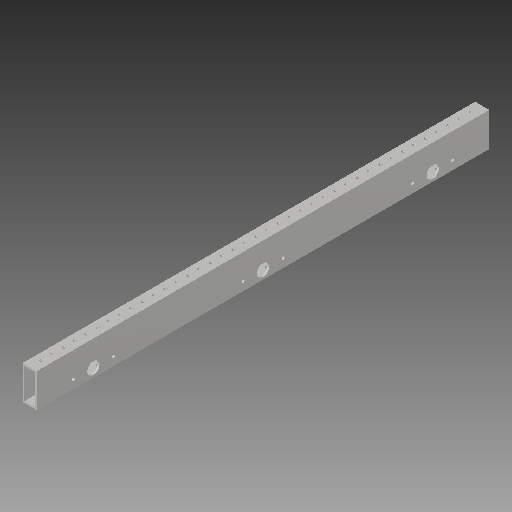
# Autodesk Inventor part: Side Extrusion
Saved by Autodesk Inventor 2019.4 (Build 234330000, 330)
## iProperties
Created: 2019-12-11
Part Number: Side Extrusion
Material: Aluminum 6061
Document SubType Name: Modeling
Designer: Mark
Mass: 988.046 g
Surface Area: 2508.19 cm^2
Volume: 365.943 cm^3
Density: 2.7 g/cm^3
Appearance: Aluminum - Flat
Author: Mark
Autodesk Inventor part; units mm, degrees
ref_plane "YZ Plane" through (0, 0, 0) normal (1, 0, 0) x (0, 1, 0)
ref_plane "XZ Plane" through (0, 0, 0) normal (0, 1, 0) x (-1, 0, 0)
ref_plane "XY Plane" through (0, 0, 0) normal (0, 0, 1) x (1, 0, 0)
sketch "Sketch1" plane through (0, 0, 0) normal (0, 0, 1) x (1, 0, 0)
  line L0 (-12.5, -30) -> (12.5, -30)
  line L1 (12.5, -30) -> (12.5, 30)
  line L2 (12.5, 30) -> (-12.5, 30)
  line L3 (-12.5, 30) -> (-12.5, -30)
  line L4 (-12.5, -30) -> (12.5, 30) construction
  line L5 (12.5, -30) -> (-12.5, 30) construction
  line L6 (-9.5, -27) -> (9.5, -27)
  line L7 (9.5, -27) -> (9.5, 27)
  line L8 (9.5, 27) -> (-9.5, 27)
  line L9 (-9.5, 27) -> (-9.5, -27)
  line L10 (-9.5, -27) -> (9.5, 27) construction
  line L11 (9.5, -27) -> (-9.5, 27) construction
  point P0 (0, 0)
  dimension "d0" = 25
  dimension "d1" = 60
  dimension "d2" = 19
  dimension "d3" = 54
  constraints: 24 end point, 4 midpoint, 4 parallel, 2 horizontal, 2 perpendicular
  measures "d0" distance of L2.end L1.end
  measures "d1" distance of L1.end L0.end
  measures "d2" distance of L8.end L7.end
  measures "d3" distance of L7.end L6.end
extrude "Extrusion1" add sketch "Sketch1" along normal blind 800
sketch "Sketch2" plane through (12.5, -30, 0) normal (1, 0, 0) x (0, 0, -1)
  circle A0 centre (-400, 15) radius 11
  circle A1 centre (-700, 15) radius 11
  circle A2 centre (-100, 15) radius 11
  line L0 (0, 60) -> (-800, 60) projected
  line L1 (-800, 0) -> (-800, 60) projected
  circle A3 centre (-700, 15) radius 35.5 construction
  circle A4 centre (-735.5, 15) radius 2.75
  circle A5 centre (-664.5, 15) radius 2.75
  line L2 (-700, 15) -> (-735.5, 15) construction
  line L3 (-700, 15) -> (-664.5, 15) construction
  line L4 (-400, 15) -> (-400, 60)
  circle A6 centre (-435.5, 15) radius 2.75
  line L5 (0, 0) -> (-800, 0) projected
  circle A7 centre (-64.5, 15) radius 2.75
  circle A8 centre (-135.5, 15) radius 2.75
  circle A9 centre (-364.5, 15) radius 2.75
  point P0 (0, 30)
  dimension "d6" = 22
  dimension "d7" = 22
  dimension "d8" = 22
  dimension "d9" = 45
  dimension "d10" = 45
  dimension "d11" = 45
  dimension "d12" = 400
  dimension "d13" = 300
  dimension "d14" = 300
  dimension "d33" = 71
  dimension "d34" = 5.5
  dimension "d35" = 5.5
  dimension "d36" = 71
  dimension "d37" = 180
  dimension "d38" = 5.5
  dimension "d39" = 35.5
  dimension "d41" = 45
  constraints: 10 centre point, 6 end point, 3 symmetric about line, 2 horizontal, 2 point on circle, 1 coincident, 1 collinear, 1 midpoint, 3 other
  measures "d6" diameter of A0
  measures "d7" diameter of A1
  measures "d8" diameter of A2
  measures "d9" distance from line of L0 L4.start
  measures "d10" distance from line of L0 A2.centre
  measures "d11" distance from line of L0 A1.centre
  measures "d12" distance from line of L1 L4.start
  measures "d13" distance of L4.start A1.centre
  measures "d14" distance of L4.start A2.centre
  measures "d33" diameter of A3
  measures "d34" diameter of A4
  measures "d35" diameter of A5
  measures "d36" distance of A5.centre L2.end
  measures "d37" angle of L2 L3
  measures "d38" diameter of A6
  measures "d39" distance of L4.start A6.centre
  measures "d41" distance from line of L0 A6.centre
extrude "Extrusion2" cut sketch "Sketch2" against normal blind 100
sketch "Sketch4" plane through (-12.5, 30, 0) normal (0, 1, 0) x (1, 0, 0)
  circle A0 centre (12.5, -20) radius 2.75
  line L0 (25, 0) -> (25, -800) projected
  line L1 (25, 0) -> (0, 0) projected
  circle A1 centre (12.5, -40) radius 2.75
  circle A2 centre (12.5, -60) radius 2.75
  circle A3 centre (12.5, -80) radius 2.75
  circle A4 centre (12.5, -100) radius 2.75
  circle A5 centre (12.5, -120) radius 2.75
  circle A6 centre (12.5, -140) radius 2.75
  circle A7 centre (12.5, -160) radius 2.75
  circle A8 centre (12.5, -180) radius 2.75
  circle A9 centre (12.5, -200) radius 2.75
  circle A10 centre (12.5, -220) radius 2.75
  circle A11 centre (12.5, -240) radius 2.75
  circle A12 centre (12.5, -260) radius 2.75
  circle A13 centre (12.5, -280) radius 2.75
  circle A14 centre (12.5, -300) radius 2.75
  circle A15 centre (12.5, -320) radius 2.75
  circle A16 centre (12.5, -340) radius 2.75
  circle A17 centre (12.5, -360) radius 2.75
  circle A18 centre (12.5, -380) radius 2.75
  circle A19 centre (12.5, -400) radius 2.75
  circle A20 centre (12.5, -420) radius 2.75
  circle A21 centre (12.5, -440) radius 2.75
  circle A22 centre (12.5, -460) radius 2.75
  circle A23 centre (12.5, -480) radius 2.75
  circle A24 centre (12.5, -500) radius 2.75
  circle A25 centre (12.5, -520) radius 2.75
  circle A26 centre (12.5, -540) radius 2.75
  circle A27 centre (12.5, -560) radius 2.75
  circle A28 centre (12.5, -580) radius 2.75
  circle A29 centre (12.5, -600) radius 2.75
  circle A30 centre (12.5, -620) radius 2.75
  circle A31 centre (12.5, -640) radius 2.75
  circle A32 centre (12.5, -660) radius 2.75
  circle A33 centre (12.5, -680) radius 2.75
  circle A34 centre (12.5, -700) radius 2.75
  circle A35 centre (12.5, -720) radius 2.75
  circle A36 centre (12.5, -740) radius 2.75
  circle A37 centre (12.5, -760) radius 2.75
  circle A38 centre (12.5, -780) radius 2.75
  circle A39 centre (12.5, -800) radius 2.75
  point P0 (12.5, 0)
  dimension "d21" = 5.5
  dimension "d22" = 12.5
  dimension "d23" = 20
  dimension "d26" = 20
  constraints: 40 centre point, 1 vertical, 78 other
  measures "d21" diameter of A0
  measures "d22" distance from line of L0 A0.centre
  measures "d23" distance from line of L1 A0.centre
  measures "d26" distance of A0.centre A1.centre
extrude "Extrusion3" cut sketch "Sketch4" against normal blind 100 contours A0 | A1 | A2 | A3 | A4 | A5 | A6 | A7 | A8 | A9 | A10 | A11 | A12 | A13 | A14 | A15 | A16 | A17 | A18 | A19 | A20 | A21 | A22 | A23 | A24 | A25 | A26 | A27 | A28 | A29 | A30 | A31 | A32 | A33 | A34 | A35 | A36 | A37 | A38
equation "\"d4\" = Length"
equation "\"d10\" = d9"
equation "\"d11\" = d9"
equation "\"d12\" = 0.5 * Length"
equation "\"d14\" = d13"
equation "\"d41\" = d9"
equation "\"Length\" = 800"
body "Solid1"
